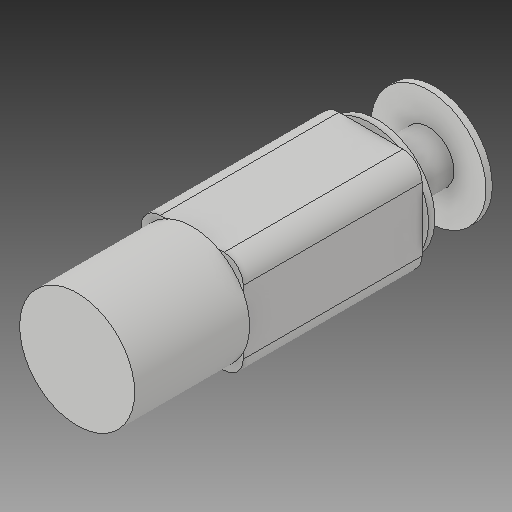
# Autodesk Inventor part: ScissorLiftMotorApproximation
Saved by Autodesk Inventor 2018 (Build 220112000, 112)
## iProperties
Created: 2020-01-25
Part Number: ScissorLiftMotorApproximation
Material: Generic
Document SubType Name: Modeling
Designer: Cooper
Density: 1 g/cm^3
Appearance: Default
Mass: 398.256 g
Surface Area: 400.58 cm^2
Volume: 398.256 cm^3
Author: Cooper
Autodesk Inventor part; units mm, degrees
ref_plane "YZ Plane" through (0, 0, 0) normal (1, 0, 0) x (0, 1, 0)
ref_plane "XZ Plane" through (0, 0, 0) normal (0, 1, 0) x (-1, 0, 0)
ref_plane "XY Plane" through (0, 0, 0) normal (0, 0, 1) x (1, 0, 0)
sketch "Sketch1" plane through (0, 0, 0) normal (0, 0, 1) x (1, 0, 0)
  circle A0 centre (0, 0) radius 28.575
  dimension "d0" = 57.15
  constraints: 1 centre point, 1 coincident
  measures "d0" diameter of A0
extrude "Extrusion1" add sketch "Sketch1" along normal blind 57.15
sketch "Sketch2" plane through (0, 0, 0) normal (0, 0, -1) x (-1, 0, 0)
  circle A0 centre (0, 0) radius 28.575 projected
  line L0 (-25.4, 25.4) -> (25.4, 25.4)
  line L1 (25.4, 25.4) -> (25.4, -25.4)
  line L2 (25.4, -25.4) -> (-25.4, -25.4)
  line L3 (-25.4, -25.4) -> (-25.4, 25.4)
  dimension "d4" = 25.4
  dimension "d5" = 25.4
  dimension "d6" = 25.4
  dimension "d7" = 25.4
  constraints: 8 end point, 2 parallel, 1 horizontal, 1 perpendicular
  measures "d4" distance from line of point (0, 0) L3
  measures "d5" distance from line of L1 point (0, 0)
  measures "d6" distance from line of point (0, 0) L0
  measures "d7" distance from line of L2 point (0, 0)
extrude "Extrusion2" add sketch "Sketch2" along normal blind 88.9 contours L1 A0 L2 L3 L0 | A0 L0 L1 | L1 L2 A0 | A0 L3 L0 | L2 L3 A0
sketch "Sketch3" plane through (0, 0, -88.9) normal (0, 0, -1) x (-1, 0, 0)
  circle A0 centre (0, 0) radius 28.575
  dimension "d10" = 57.15
  constraints: 1 centre point, 1 coincident
  measures "d10" diameter of A0
extrude "Extrusion3" add sketch "Sketch3" along normal blind 3.175
sketch "Sketch4" plane through (0, 0, -92.075) normal (0, 0, -1) x (-1, 0, 0)
  circle A0 centre (0, 0) radius 12.7
  dimension "d13" = 25.4
  constraints: 1 centre point, 1 coincident
  measures "d13" diameter of A0
extrude "Extrusion4" add sketch "Sketch4" along normal blind 25.4
sketch "Sketch5" plane through (0, 0, -117.475) normal (0, 0, -1) x (-1, 0, 0)
  circle A0 centre (0, 0) radius 28.575
  dimension "d16" = 57.15
  constraints: 1 centre point, 1 coincident
  measures "d16" diameter of A0
extrude "Extrusion5" add sketch "Sketch5" along normal blind 3.175
fillet "Fillet1" radius 9.525 4 edges at (25.4, 25.4, -44.45) (-25.4, 25.4, -44.45) (25.4, -25.4, -44.45) (-25.4, -25.4, -44.45)
equation "\"d4\" = d5"
equation "\"d7\" = d6"
body "Solid1"
